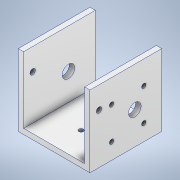
# Autodesk Inventor part: hand
Saved by Autodesk Inventor 2022 (Build 260153000, 153)
## iProperties
Created: 2022-04-20
Part Number: hand
Material: アルミニウム 6061
Document SubType Name: Modeling
Designer: Yazawa
Density: 2.7 g/cm^3
Appearance: アルミニウム - フラット
Author: Yazawa
Autodesk Inventor part; units mm, degrees
ref_plane "YZ Plane" through (0, 0, 0) normal (1, 0, 0) x (0, 1, 0)
ref_plane "XZ Plane" through (0, 0, 0) normal (0, 1, 0) x (-1, 0, 0)
ref_plane "XY Plane" through (0, 0, 0) normal (0, 0, 1) x (1, 0, 0)
sketch "スケッチ1" plane through (0, 0, 0) normal (0, 1, 0) x (-1, 0, 0)
  line L0 (20, -20) -> (-20, -20)
  line L1 (-20, -20) -> (-20, 20)
  line L2 (-20, 20) -> (20, 20)
  line L3 (20, 20) -> (20, -20)
  line L4 (-20, 20) -> (20, -20) construction
  line L5 (-20, -20) -> (20, 20) construction
  point P0 (0, 0)
  point P1 (0, 0)
  dimension "d0" = 40
  dimension "d1" = 40
  constraints: 12 end point, 2 midpoint, 2 parallel, 1 coincident, 1 horizontal, 1 perpendicular
  measures "d0" distance of L1.end L2.end
  measures "d1" distance of L0.end L1.end
extrude "押し出し1" add sketch "スケッチ1" along normal blind 3
sketch "スケッチ2" plane through (0, 3, 0) normal (0, 1, 0) x (1, 0, 0)
  line L0 (-20, -20) -> (20, -20) projected
  line L1 (20, -20) -> (20, 20) projected
  line L2 (20, 20) -> (-20, 20) projected
  line L3 (-20, 20) -> (-20, -20) projected
  line L4 (-20, -20) -> (20, -20) projected
  line L5 (-20, -20) -> (-17, -20)
  line L6 (-17, -20) -> (-17, 20)
  line L7 (-17, 20) -> (-20, 20)
  line L8 (-20, 20) -> (-20, -20)
  line L9 (20, -20) -> (20, 20) projected
  line L10 (20, -20) -> (17, -20)
  line L11 (17, -20) -> (17, 20)
  line L12 (17, 20) -> (20, 20)
  line L13 (20, 20) -> (20, -20)
  line L14 (20, 20) -> (-20, 20) projected
  point P0 (0, 0)
  point P1 (-17, 20)
  dimension "d4" = 3
  dimension "d5" = 3
  constraints: 16 end point, 4 parallel, 2 collinear, 2 horizontal, 2 perpendicular
  measures "d4" distance of L7.end L6.end
  measures "d5" distance of L11.end L12.end
extrude "押し出し2" add sketch "スケッチ2" along normal blind 40 from surface at -3 contours L3 L2 L6 L0 | L11 L2 L1 L0
sketch "スケッチ3" plane through (20, 0, 20) normal (1, 0, 0) x (0, 0, -1)
  line L0 (0, 3) -> (40, 3) projected
  line L1 (25, 18) -> (40, 18) construction
  line L2 (40, 40) -> (40, 3) construction
  line L3 (25, 18) -> (-0.0782, 18) construction
  point P0 (20, 0)
  dimension "d8" = 15
  dimension "d50" = 15
  constraints: 4 end point, 2 point on line, 1 horizontal
  measures "d8" distance from line of L0 L1.start
  measures "d50" distance of L1.start L1.end
hole "穴1" at (20, 18, -5) direction (-1, 0, 0) diameter 7 end through all
sketch "スケッチ5" plane through (20, 0, 20) normal (1, 0, 0) x (0, 0, -1)
  line L0 (0, 0) -> (0, 40) projected
  line L1 (0, 0) -> (40, 0) projected
  line L2 (36, 33) -> (6, 33)
  line L3 (6, 33) -> (6, 3)
  line L4 (6, 3) -> (36, 3)
  line L5 (36, 3) -> (36, 33)
  line L6 (36, 33) -> (6, 3) construction
  line L7 (36, 3) -> (6, 33) construction
  line L8 (36, 18) -> (6, 18)
  circle A0 centre (25, 18) radius 3.5 projected
  point P0 (20, 0)
  point P1 (21, 18)
  point P2 (30, 27)
  point P3 (12, 27)
  point P4 (21, 18)
  point P5 (12, 9)
  point P6 (21, 18)
  point P7 (30, 9)
  point P8 (21, 18)
  point P9 (30, 27)
  dimension "d20" = 30
  dimension "d21" = 30
  dimension "d23" = 6
  dimension "d24" = 6
  dimension "d27" = 360
  dimension "d40" = 4
  constraints: 14 end point, 3 coincident, 3 midpoint, 2 parallel, 1 horizontal, 1 horizontal alignment, 1 perpendicular, 1 symmetric about line, 7 other
  measures "d20" distance of L4.end L3.end
  measures "d21" distance of L3.end L2.end
  measures "d23" distance from line of L5 point (30, 27)
  measures "d24" distance from line of L2 point (30, 27)
  measures "d40" distance of point (21, 18) point (25, 18)
hole "穴2" at (20, 27, -10) at (20, 9, -10) at (20, 27, 8) at (20, 9, 8) direction (-1, 0, 0) diameter 2.459 depth 3 thread size "M3x0.5" class "6H" standard "ISO Metric profile"
sketch "スケッチ6" plane through (0, 3, 0) normal (0, 1, 0) x (1, 0, 0)
  line L0 (17, 20) -> (-17, 20) projected
  point P0 (0, 0)
  point P1 (0, 15)
  point P2 (0, -5)
  point P3 (0, 20)
  dimension "d41" = 5
  dimension "d42" = 20
  constraints: 2 vertical alignment, 1 midpoint
  measures "d41" distance from line of L0 point (0, 15)
  measures "d42" distance of point (0, -5) point (0, 15)
hole "穴3" at (0, 3, -15) at (0, 3, 5) direction (0, -1, 0) diameter 2.459 depth 3 thread size "M3x0.5" class "6H" standard "ISO Metric profile"
sketch "スケッチ7" plane through (20, 0, 20) normal (1, 0, 0) x (0, 0, -1)
  circle A0 centre (25, 18) radius 3.5 projected
  line L0 (25, 18) -> (-12.3311, 18)
  line L1 (-6.2752, 36.0567) -> (25, 18)
  circle A1 centre (5, 27.815) radius 1.5
  line L2 (0, 0) -> (0, 40) projected
  point P0 (20, 0)
  dimension "d51" = 30
  dimension "d52" = 3
  dimension "d53" = 5
  constraints: 4 end point, 1 centre point, 1 horizontal, 1 tangent
  measures "d51" angle of L1 L0
  measures "d52" diameter of A1
  measures "d53" distance from line of L2 A1.centre
extrude "押し出し4" cut sketch "スケッチ7" against normal up to surface (40 mm away) contours A1
equation "\"d54\" = d53"
